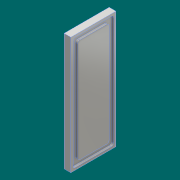
# Autodesk Inventor part: plateEnd
Saved by Autodesk Inventor 2016 (Build 200138000, 138)
## iProperties
Created: 2016-07-15
Part Number: plateEnd
Material: Aluminum 6061
Document SubType Name: Modeling
Designer: Jonathan
Density: 2.7 g/cm^3
Appearance: Aluminum - Flat
Author: Jonathan
Autodesk Inventor part; units mm, degrees
ref_plane "YZ Plane" through (0, 0, 0) normal (1, 0, 0) x (0, 1, 0)
ref_plane "XZ Plane" through (0, 0, 0) normal (0, 1, 0) x (-1, 0, 0)
ref_plane "XY Plane" through (0, 0, 0) normal (0, 0, 1) x (1, 0, 0)
sketch "Sketch1" plane through (0, 0, 0) normal (1, 0, 0) x (0, 1, 0)
  line L0 (31.75, 82.55) -> (-31.75, 82.55)
  line L1 (-31.75, 82.55) -> (-31.75, -82.55)
  line L2 (-31.75, -82.55) -> (31.75, -82.55)
  line L3 (31.75, -82.55) -> (31.75, 82.55)
  point P0 (0, 0)
  point P1 (31.75, 0)
  point P2 (0, 82.55)
  dimension "d0" = 165.1
  dimension "d1" = 63.5
  constraints: 8 end point, 2 midpoint, 2 parallel, 1 horizontal, 1 horizontal alignment, 1 perpendicular, 1 vertical alignment
  measures "d0" distance of L2.end L0.start
  measures "d1" distance of L1.end L2.end
extrude "Extrusion1" add sketch "Sketch1" along normal blind 9.525
sketch "Sketch3" plane through (9.525, 0, 0) normal (1, 0, 0) x (0, 0, -1)
  line L0 (72.898, -22.098) -> (-72.898, -22.098)
  line L1 (-72.898, -22.098) -> (-72.898, 22.098)
  line L2 (-72.898, 22.098) -> (72.898, 22.098)
  line L3 (72.898, 22.098) -> (72.898, -22.098)
  line L4 (72.898, -22.098) -> (-72.898, 22.098) construction
  line L5 (-72.898, -22.098) -> (72.898, 22.098) construction
  line L6 (79.375, -28.575) -> (-79.375, -28.575)
  line L7 (-79.375, -28.575) -> (-79.375, 28.575)
  line L8 (-79.375, 28.575) -> (79.375, 28.575)
  line L9 (79.375, 28.575) -> (79.375, -28.575)
  line L10 (79.375, -28.575) -> (-79.375, 28.575) construction
  line L11 (-79.375, -28.575) -> (79.375, 28.575) construction
  point P0 (0, 0)
  point P1 (0, 0)
  point P2 (0, 0)
  dimension "d16" = 145.796
  dimension "d17" = 44.196
  dimension "d18" = 6.477
  dimension "d19" = 6.477
  constraints: 24 end point, 5 midpoint, 4 parallel, 2 horizontal, 2 perpendicular, 1 coincident
  measures "d16" distance of L1.end L2.end
  measures "d17" distance between parallel lines of L0 L2
  measures "d18" distance between parallel lines of L8 L2
  measures "d19" distance between parallel lines of L7 L1
extrude "Extrusion3" cut sketch "Sketch3" against normal blind 3.175
fillet "Fillet1" radius 3.175 8 edges at (7.9375, -28.575, 79.375) (7.9375, 28.575, 79.375) (7.9375, 28.575, -79.375) (7.9375, -28.575, -79.375) (7.9375, -22.098, 72.898) (7.9375, 22.098, 72.898) (7.9375, 22.098, -72.898) (7.9375, -22.098, -72.898)
equation "\"d0\" = tubeWidth + 2 * plateOverhang"
equation "\"d1\" = tubeHeight + 2 * plateOverhang"
equation "\"d2\" = blankCapThickness"
equation "\"d16\" = -2 * tubeWallThickness + tubeWidth - 2 * tubePlateClearance"
equation "\"d17\" = -2 * tubeWallThickness + tubeHeight - 2 * tubePlateClearance"
equation "\"d18\" = tubeWallThickness + tubePlateClearance + moatWidth"
equation "\"d19\" = tubeWallThickness + tubePlateClearance + moatWidth"
equation "\"d12\" = moatDepth"
equation "\"tubeHeight\" = 50.8"
equation "\"tubeWidth\" = 152.4"
equation "\"tubeLength\" = 304.8"
equation "\"tubeWallThickness\" = 3.175"
equation "\"plateOverhang\" = 6.35"
equation "\"moatWidth\" = 3.175"
equation "\"tubePlateClearance\" = 0.127"
equation "\"moatDepth\" = 3.175"
equation "\"blankCapThickness\" = 9.525"
equation "\"fiberClearance\" = 0"
equation "\"oRingID\" = 22.2504"
equation "\"fiberDiameter\" = 1"
equation "\"sensorHolderThickness\" = 12.7"
equation "\"oRingGrooveWidth\" = 2.54"
equation "\"longHoleSpacing\" = 30.48"
equation "\"sensorHolderDiameter\" = 50.8"
equation "\"shortHoleSpacing\" = 21.59"
equation "\"glassTubeClearance\" = 0.19844"
equation "\"glassTubeDiameter\" = 12.7"
equation "\"sensorCapThickness\" = 12.7"
equation "\"oRingGrooveDepth\" = 1.2446"
equation "\"glassTubeID\" = 7.874"
equation "\"glassTubeLength\" = 279.4"
equation "\"sensorBoardHoleSpacing\" = 19"
body "Solid1"
